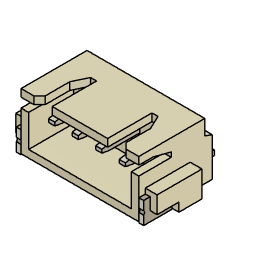
JST-XH SMD Parametric (Autodesk Fusion 360 design; units mm, degrees)
Autodesk Fusion 360 part; units mm, degrees
sketch "Top Ref" plane through (0, 0, 0) normal (0, 0, 1) x (1, 0, 0)
  line L0 (6.25, 0) -> (-6.25, 0)
  line L1 (-6.25, 0) -> (-6.25, -7.8)
  line L2 (-6.25, -7.8) -> (6.25, -7.8)
  line L3 (6.25, -7.8) -> (6.25, 0)
  line L4 (6.25, 0) -> (-6.25, -7.8) construction
  line L5 (-6.25, 0) -> (6.25, -7.8) construction
  line L6 (6.25, -2.35) -> (7.5, -2.35)
  line L7 (7.5, -2.35) -> (7.5, -7.11)
  line L8 (7.5, -7.11) -> (6.25, -7.11)
  line L9 (6.25, -7.11) -> (6.25, -2.35)
  line L10 (0, 0) -> (0, -7.8) construction
  line L11 (-4.07, 0) -> (-4.07, 1.65)
  line L12 (-4.07, 1.65) -> (-3.9378, 2.4)
  line L13 (-3.9378, 2.4) -> (-3.5622, 2.4)
  line L14 (-3.5622, 2.4) -> (-3.43, 1.65)
  line L15 (-3.43, 1.65) -> (-3.43, 0)
  line L16 (-3.75, 2.4) -> (-3.75, 0) construction
  line L17 (-4.07, 1.65) -> (-3.43, 1.65) construction
  line L18 (-6.25, -2.35) -> (-7.5, -2.35)
  line L19 (-7.5, -2.35) -> (-7.5, -7.11)
  line L20 (-7.5, -7.11) -> (-6.25, -7.11)
  line L21 (6.75, -7.11) -> (6.75, -7.8)
  line L22 (6.75, -7.8) -> (6.25, -7.8)
  line L23 (-6.75, -7.11) -> (-6.75, -7.8)
  line L24 (-6.75, -7.8) -> (-6.25, -7.8)
  line L25 (-4.89, -7.8) -> (-4.29, -7.2)
  line L26 (-4.29, -7.2) -> (-4.29, -4.6)
  line L27 (-4.29, -4.6) -> (-3.58, -3.1)
  line L28 (-3.58, -3.1) -> (-2.94, -3.1)
  line L29 (-2.94, -3.1) -> (-2.94, -7.8)
  line L30 (4.89, -7.8) -> (4.29, -7.2)
  line L31 (4.29, -7.2) -> (4.29, -4.6)
  line L32 (4.29, -4.6) -> (3.58, -3.1)
  line L33 (3.58, -3.1) -> (2.94, -3.1)
  line L34 (2.94, -3.1) -> (2.94, -7.8)
  point P0 (0, -3.9)
  point P1 (-3.75, 1.65)
  dimension "d5" = 12.5
  dimension "d6" = 7.5
  dimension "d7" = 4.76
  dimension "d8" = 0.69
  dimension "d9" = 7.8
  dimension "d10" = 0.64
  dimension "d11" = 2.4
  dimension "d12" = 3.75
  dimension "d13" = 80
  dimension "d14" = 0.75
  dimension "d16" = 0.5
  dimension "d17" = 1.35
  dimension "d18" = 4.7
  dimension "d19" = 0.64
  dimension "d20" = 1.5
  dimension "d21" = 45
  dimension "d22" = 1.96
  dimension "d23" = 0.6
  constraint horizontal L0
  constraint perpendicular L0 L1
  constraint parallel L0 L2
  constraint parallel L1 L3
  constraint coincident L4 P0
  constraint coincident L5 P0
  constraint midpoint L10.start L0
  constraint horizontal L6
  constraint vertical L7
  constraint horizontal L8
  constraint vertical L9
  constraint coincident L3 L6.start
  constraint coincident L10.start origin
  constraint midpoint L2 L10.end
  constraint coincident L0 L11.start
  constraint perpendicular L0 L11
  constraint parallel L0 L13
  constraint coincident L0 L15.end
  constraint perpendicular L0 L15
  constraint midpoint L13 L16.start
  constraint coincident L0 L16.end
  constraint perpendicular L0 L16
  constraint horizontal L11.end L14.end
  constraint perpendicular L15 L17
  constraint coincident L16 P1
  constraint midpoint L17 P1
  constraint coincident L1 L18.start
  constraint perpendicular L1 L18
  constraint perpendicular L18 L19
  constraint coincident L1 L20.end
  constraint perpendicular L1 L20
  constraint equal L6 L18
  constraint equal L7 L19
  constraint horizontal L8.end L20.end
  constraint coincident L8 L21.start
  constraint perpendicular L8 L21
  constraint perpendicular L21 L22
  constraint coincident L20 L23.start
  constraint perpendicular L20 L23
  constraint perpendicular L23 L24
  constraint equal L22 L24
  constraint coincident L2 L25.start
  constraint perpendicular L2 L26
  constraint perpendicular L26 L28
  constraint coincident L2 L29.end
  constraint perpendicular L2 L29
  constraint symmetric L10 L25.start L30.start
  constraint symmetric L10 L25.end L30.end
  constraint symmetric L10 L26.end L31.end
  constraint symmetric L10 L27.end L32.end
  constraint symmetric L10 L28.end L33.end
  constraint symmetric L10 L29.end L34.end
  constraint coincident L2.end L3.start
  constraint coincident L1.end L2.start
  measures "d5" distance of L1.end L2.end
  measures "d6" distance of L10.start L7
  measures "d7" distance of L6.end L7.end
  measures "d8" distance of L2.end L8
  measures "d9" distance of L0.end L1.end
  measures "d10" distance of L11.end L14.end
  measures "d11" distance of L16.start L16.end
  measures "d12" distance of L10.start L16.end
  measures "d13" angle of L14 L17
  measures "d14" distance of L13 L14.end
  measures "d16" distance of L21.end L2.end
  measures "d17" distance of L26 L29
  measures "d18" distance of L2 L28
  measures "d19" distance of L27.end L28.end
  measures "d20" distance of L26.end L28
  measures "d21" angle of L2 L25
  measures "d22" distance of L1 L26
  measures "d23" distance of L2 L25.end
sketch "Side Ref" plane through (0, 0, 0) normal (1, 0, 0) x (0, 1, 0)
  line L0 (0, 0) -> (0, 6)
  line L1 (0, 6) -> (-7.8, 6)
  line L2 (-7.8, 6) -> (-7.8, 0)
  line L3 (-7.8, 0) -> (0, 0)
  line L4 (0, 4.1) -> (-0.8, 4.395)
  line L5 (-0.8, 4.395) -> (-0.8, 6)
  line L6 (-0.8, 5.47) -> (-1.33, 5.47)
  line L7 (-1.33, 5.47) -> (-1.33, 4.395)
  line L8 (-1.33, 4.395) -> (-0.9, 4.395)
  line L9 (-0.9, 4.395) -> (-0.9, 3.145)
  line L10 (-0.9, 3.145) -> (-1.5, 3.145)
  line L11 (-1.5, 3.145) -> (-1.5, 1.12)
  line L12 (-1.5, 1.12) -> (0, 1.12)
  line L13 (-7.8, 5.2) -> (-3.03, 5.2)
  line L14 (-6.3, 5.2) -> (-4.35, 4.7)
  line L15 (-4.35, 4.7) -> (-4.35, 4.2)
  line L16 (-4.35, 4.2) -> (-7.8, 4.2)
  line L17 (-3.03, 5.2) -> (-3.03, 0.8)
  line L18 (-3.03, 0.8) -> (-7.8, 0.8)
  line L19 (-4.35, 4.7) -> (-4.35, 5.2) construction
  line L20 (-3.03, 4.09) -> (-6.25, 4.09)
  line L21 (-6.25, 4.09) -> (-7.05, 3.9489)
  line L22 (-7.05, 3.9489) -> (-7.05, 3.5911)
  line L23 (-7.05, 3.5911) -> (-6.25, 3.45)
  line L24 (-6.25, 3.45) -> (-3.03, 3.45)
  line L25 (-7.05, 3.77) -> (-3.03, 3.77) construction
  point P0 (-1.065, 5.47)
  point P1 (-0.9, 3.77)
  dimension "d24" = 6
  dimension "d25" = 7.8
  dimension "d26" = 7
  dimension "d27" = 1.9
  dimension "d29" = 1.12
  dimension "d30" = 1.5
  dimension "d31" = 0.53
  dimension "d32" = 0.53
  dimension "d34" = 1.25
  dimension "d36" = 0.1
  dimension "d60" = 0.8
  dimension "d61" = 0.8
  dimension "d62" = 4.77
  dimension "d63" = 3.45
  dimension "d64" = 1.5
  dimension "d65" = 1
  dimension "d66" = 0.8
  dimension "d67" = 10
  dimension "d68" = 0.64
  dimension "d69" = 0.75
  dimension "d70" = 2.55
  constraint coincident L0.start L3.end
  constraint vertical L0
  constraint perpendicular L0 L1
  constraint perpendicular L1 L2
  constraint horizontal L3
  constraint coincident L0 L4.start
  constraint coincident L1 L5.end
  constraint perpendicular L1 L5
  constraint coincident L5 L6.start
  constraint perpendicular L5 L6
  constraint perpendicular L6 L7
  constraint perpendicular L7 L8
  constraint perpendicular L8 L9
  constraint perpendicular L7 L10
  constraint perpendicular L3 L11
  constraint coincident L0 L12.end
  constraint perpendicular L0 L12
  constraint midpoint L6 P0
  constraint horizontal L4.end L8.end
  constraint coincident L2 L13.start
  constraint perpendicular L2 L13
  constraint perpendicular L13 L15
  constraint coincident L2 L16.end
  constraint perpendicular L2 L16
  constraint perpendicular L13 L17
  constraint coincident L2 L18.end
  constraint perpendicular L2 L18
  constraint coincident L14.start L13
  constraint coincident L13 L19.end
  constraint perpendicular L13 L19
  constraint equal L15 L19
  constraint coincident L17 L20.start
  constraint perpendicular L17 L20
  constraint perpendicular L20 L22
  constraint coincident L17 L24.end
  constraint perpendicular L17 L24
  constraint midpoint L22 L25.start
  constraint coincident L17 L25.end
  constraint perpendicular L17 L25
  constraint vertical L20.end L23.end
  constraint equal L21 L23
  constraint midpoint L9 P1
  constraint horizontal L25.end P1
  measures "d24" distance of L0.start L0.end
  measures "d25" distance of L0.end L1.end
  measures "d26" distance of L1.end L5.end
  measures "d27" distance of L0.end L4.start
  measures "d29" distance of L12 L0.start
  measures "d30" distance of L11.end L12.end
  measures "d31" distance of L1 L6
  measures "d32" distance of L6.start L6.end
  measures "d34" distance of L8.end L9.end
  measures "d36" distance of L4.end L8.end
  measures "d60" distance of L1 L13
  measures "d61" distance of L3 L18
  measures "d62" distance of L13.start L13.end
  measures "d63" distance of L15.end L16.end
  measures "d64" distance of L13.start L14.start
  measures "d65" distance of L13 L16
  measures "d66" horizontal distance of L20.end L21.end
  measures "d67" angle of L20 L21
  measures "d68" distance of L20 L24
  measures "d69" distance of L2 L25.start
  measures "d70" distance of L1 L23.end
extrude "Extrude1" add sketch "Side Ref" along normal mid plane 12.5 contours L0 L1 L2 L3 L5 L6 L7 L8 L9 L10 L11 L12 L13 L17 L18 | L2 L13 L14 L15 L16 L17 L18 L20 L21 L22 L23 L24 | L2 L13 L14 L15 L16 | L17 L20 L21 L22 L23 L24 makes body 1
ref_plane "WorkPlane1" through (-3.75, 1.2, 0) normal (-1, 0, 0) x (0, -1, 0)
extrude "Extrude2" add sketch "Side Ref" against normal blind 0.82 from surface at 6.25 contours L0 L1 L2 L3 L5 L6 L7 L8 L9 L10 L11 L12 L13 L17 L18 | L0 L4 L5 L6 L7 L8 L9 L10 L11 L12 | L2 L13 L14 L15 L16 L17 L18 L20 L21 L22 L23 L24 | L2 L13 L14 L15 L16 | L17 L20 L21 L22 L23 L24 bodies 1
extrude "Extrude3" add sketch "Side Ref" along normal blind 0.82 from surface at -6.25 contours L0 L1 L2 L3 L5 L6 L7 L8 L9 L10 L11 L12 L13 L17 L18 | L0 L4 L5 L6 L7 L8 L9 L10 L11 L12 | L2 L13 L14 L15 L16 L17 L18 L20 L21 L22 L23 L24 | L2 L13 L14 L15 L16 | L17 L20 L21 L22 L23 L24 bodies 1
extrude "Extrude6" cut sketch "Side Ref" along normal mid plane 10.9 contours L2 L13 L14 L15 L16 L17 L18 L20 L21 L22 L23 L24 | L2 L13 L14 L15 L16 | L17 L20 L21 L22 L23 L24 bodies 1
extrude "Extrude7" cut sketch "Side Ref" along normal mid plane 12.5 contours L2 L13 L14 L15 L16 bodies 1
extrude "Extrude8" cut sketch "Top Ref" along normal blind 6 from surface at 1 contours L2 L30 L31 L32 L33 L34 | L2 L25 L26 L27 L28 L29 bodies 1
sketch "Pin Side" plane through (-3.75, 0, 0) normal (-1, 0, 0) x (0, -1, 0)
  line L0 (-2.4, 0) -> (0, 0) construction
  line L1 (-2.4, -0.1) -> (0.64, -0.1)
  line L2 (-2.4, -0.1) -> (-2.4, 0.54)
  line L3 (-2.4, 0.54) -> (0, 0.54)
  line L4 (0.64, -0.1) -> (0.64, 3.45)
  line L5 (0, 0.54) -> (0, 4.09)
  line L6 (0.9, 4.395) -> (0.9, 3.145) construction
  line L7 (0.9, 4.09) -> (0.9, 3.45)
  line L8 (0.9, 4.09) -> (0, 4.09)
  line L9 (0.9, 3.45) -> (0.64, 3.45)
  line L10 (0.64, 3.45) -> (0, 3.45) construction
  line L11 (-2.4, 0.4078) -> (-1.65, 0.54)
  arc A0 (0.2, 4.09) -> (0, 3.89) centre (0.2, 3.89) ccw
  arc A1 (-0.1, 0.54) -> (0, 0.64) centre (-0.1, 0.64) ccw
  line L12 (6.25, 4.09) -> (7.05, 3.9489)
  line L13 (7.05, 3.9489) -> (7.05, 3.5911)
  line L14 (7.05, 3.5911) -> (6.25, 3.45)
  line L15 (6.25, 3.45) -> (3.03, 3.45)
  line L16 (3.03, 4.09) -> (6.25, 4.09)
  line L17 (3.03, 4.09) -> (3.03, 3.45)
  line L18 (3.03, 4.09) -> (0.9, 4.09)
  line L19 (3.03, 3.45) -> (0.9, 3.45)
  point P0 (0.9, 3.77)
  point P1 (-1.65, 0)
  dimension "d46" = 0.1
  dimension "d47" = 0.64
  dimension "d48" = 10
  dimension "d49" = 0.2
  dimension "d50" = 0.1
  constraint horizontal L1
  constraint vertical L0.start L1.start
  constraint perpendicular L0 L2
  constraint perpendicular L2 L3
  constraint perpendicular L1 L4
  constraint perpendicular L3 L5
  constraint midpoint L6 P0
  constraint coincident L6 L7.start
  constraint coincident L6 L7.end
  constraint parallel L6 L7
  constraint midpoint P0 L7
  constraint horizontal L8
  constraint horizontal L9
  constraint equal L2 L7
  constraint coincident L5 L10.end
  constraint perpendicular L5 L10
  constraint equal L2 L10
  constraint vertical L3.end L0.end
  constraint coincident L2 L11.start
  constraint coincident L3 L11.end
  constraint vertical P1 L11.end
  constraint tangent L8 A0
  constraint coincident L5 A0.end
  constraint coincident L8 A0.start
  constraint tangent L5 A0
  constraint coincident L3 A1.start
  constraint coincident L5 A1.end
  constraint tangent L5 A1
  constraint tangent L3 A1
  constraint coincident L16.start L17.start
  constraint coincident L15.end L17.end
  constraint coincident L7.start L8.start
  constraint coincident L7.end L9.start
  measures "d46" distance of L0.start L1.start
  measures "d47" distance of L1.start L2.end
  measures "d48" angle of L3 L11
  measures "d49" radius of A0
  measures "d50" radius of A1
extrude "Extrude4" cut sketch "Pin Side" along normal mid plane 0.66 contours L1 L2 L3 L4 L5 L7 L8 L9 L11 A0 | L7 L17 L18 L19 | L3 L5 A1 | L12 L13 L14 L15 L16 L17 | L5 L8 A0 bodies 1
extrude "Extrude5" add sketch "Pin Side" along normal mid plane 0.65 separate body contours L1 L2 L3 L4 L5 L7 L8 L9 L11 A0 | L7 L17 L18 L19 | L3 L5 A1 | L12 L13 L14 L15 L16 L17 makes body 2
pattern_linear "R-Pattern1" count 4 spacing 2.5 along (1, 0, 0) of "Extrude4"
pattern_linear "R-Pattern3" count 4 spacing 2.5 along (1, 0, 0) of bodies 2 makes body 3 at (-1.575, -2.3633, 3.8767) makes body 4 at (0.925, -2.3633, 3.8767) makes body 5 at (3.425, -2.3633, 3.8767)
sketch "Side Anchors" plane through (0, 0, 0) normal (1, 0, 0) x (0, 1, 0)
  line L0 (-7.8, 6) -> (-7.8, 0) construction
  line L1 (-7.8, 0) -> (0, 0) construction
  line L2 (-2.35, 0) -> (-2.35, 2.75)
  line L3 (-2.35, 2.75) -> (-7.11, 2.75)
  line L4 (-7.11, 2.75) -> (-7.11, 0.93)
  line L5 (-7.11, 0.93) -> (-4.8, 0.93)
  line L6 (-7.8, -0.1) -> (-7.8, 2.21)
  line L7 (-7.8, 2.21) -> (-4.8, 2.21)
  line L8 (-4.8, 2.21) -> (-4.8, -0.1)
  line L9 (-4.8, -0.1) -> (-7.8, -0.1)
  line L10 (-2.35, 0) -> (-4.8, 0)
  arc A0 (-7.8, 0.855) -> (-7.8, 1.255) centre (-7.95, 1.055) ccw
  point P0 (-7.8, 0)
  point P1 (-7.11, 0)
  point P2 (-2.35, 0)
  point P3 (-7.8, 1.055)
  dimension "d79" = 2.75
  dimension "d80" = 1.82
  dimension "d81" = 2.31
  dimension "d82" = 0.1
  dimension "d83" = 3
  dimension "d95" = 0.25
  dimension "d96" = 0.15
  constraint coincident P2 L2.start
  constraint perpendicular L1 L2
  constraint perpendicular L0 L3
  constraint perpendicular L3 L4
  constraint perpendicular L0 L5
  constraint vertical P1 L4.end
  constraint vertical L6
  constraint perpendicular L0 L7
  constraint perpendicular L7 L8
  constraint perpendicular L8 L9
  constraint coincident L6.start L9.end
  constraint coincident L5.end L8
  constraint coincident L8 L10.end
  constraint coincident L1 L10.end
  constraint coincident P0 L6
  constraint coincident L0 A0.start
  constraint coincident L6 P3
  constraint midpoint L6 P3
  constraint horizontal A0.centre P3
  constraint coincident L6 A0.end
  measures "d79" distance of P2 L2.end
  measures "d80" distance of L3.end L4.end
  measures "d81" distance of L6.start L6.end
  measures "d82" vertical distance of P0 L6.start
  measures "d83" distance of L8.end L6.start
  measures "d95" radius of A0
  measures "d96" distance of A0.centre P3
extrude "Extrude9" add sketch "Side Anchors" along normal blind 1.25 from surface at 6.25 contours L2 L3 L4 L7 L8 L10 | L4 L5 L7 L8 bodies 1 2
extrude "Extrude10" cut sketch "Side Anchors" along normal blind 0.52 from surface at 6.25 contours L4 L5 L6 L7 L8 L9 A0 | L4 L5 L7 L8 | L6 A0 bodies 2 1
extrude "Extrude11" add sketch "Side Anchors" along normal blind 0.5 from surface at 6.26 separate body contours L4 L5 L6 L7 L8 L9 A0 | L4 L5 L7 L8 makes body 6
mirror "Mirror1" about plane through (0, 0, 0) normal (1, 0, 0) of "Extrude9", "Extrude10"
mirror "Mirror3" about plane through (0, 0, 0) normal (1, 0, 0) of bodies 6 makes body 7
ref_plane "WorkPlane2" through (-3.75, 0.88, -0.1) normal (0, 0, 1) x (0, -1, 0)
sketch "Footprint Reference" plane through (0, 0, -0.1) normal (0, 0, 1) x (1, 0, 0)
  line L0 (6.25, -7.8) -> (6.25, 0) construction
  line L1 (6.25, 0) -> (-6.25, 0) construction
  line L2 (-6.25, -7.8) -> (6.25, -7.8) construction
  line L3 (-6.25, 0) -> (-6.25, -7.8) construction
  line L4 (6.26, -7.8) -> (6.26, -4.8) construction
  line L5 (6.26, -4.8) -> (6.76, -4.8) construction
  line L6 (6.76, -4.8) -> (6.76, -7.8) construction
  line L7 (6.76, -7.8) -> (6.26, -7.8) construction
  line L8 (-6.26, -4.8) -> (-6.26, -7.8) construction
  line L9 (-6.26, -7.8) -> (-6.76, -7.8) construction
  line L10 (-6.76, -7.8) -> (-6.76, -4.8) construction
  line L11 (-6.76, -4.8) -> (-6.26, -4.8) construction
  line L12 (-3.425, -0.64) -> (-4.075, -0.64) construction
  line L13 (-4.075, -0.64) -> (-4.075, 2.4) construction
  line L14 (-4.075, 2.4) -> (-3.425, 2.4) construction
  line L15 (-3.425, 2.4) -> (-3.425, -0.64) construction
  line L16 (-3.225, -0.84) -> (-4.275, -0.84)
  line L17 (-4.275, -0.84) -> (-4.275, 2.6)
  line L18 (-4.275, 2.6) -> (-3.225, 2.6)
  line L19 (-3.225, 2.6) -> (-3.225, -0.84)
  line L20 (-6.06, -8) -> (-6.96, -8)
  line L21 (-6.96, -8) -> (-6.96, -4.6)
  line L22 (-6.96, -4.6) -> (-6.06, -4.6)
  line L23 (-6.06, -4.6) -> (-6.06, -8)
  line L24 (6.96, -8) -> (6.06, -8)
  line L25 (6.06, -8) -> (6.06, -4.6)
  line L26 (6.06, -4.6) -> (6.96, -4.6)
  line L27 (6.96, -4.6) -> (6.96, -8)
  line L28 (-4.275, 2.6) -> (-3.225, -0.84) construction
  line L29 (-3.225, 2.6) -> (-4.275, -0.84) construction
  line L30 (-6.96, -4.6) -> (-6.06, -8) construction
  line L31 (-6.96, -8) -> (-6.06, -4.6) construction
  line L32 (6.96, -4.6) -> (6.06, -8) construction
  line L33 (6.96, -8) -> (6.06, -4.6) construction
  line L34 (-0.725, -0.84) -> (-1.775, -0.84)
  line L35 (-1.775, -0.84) -> (-1.775, 2.6)
  line L36 (-0.725, 2.6) -> (-0.725, -0.84)
  line L37 (-1.775, 2.6) -> (-0.725, 2.6)
  line L38 (-0.725, 2.6) -> (-1.775, -0.84) construction
  line L39 (-1.775, 2.6) -> (-0.725, -0.84) construction
  line L40 (1.775, -0.84) -> (0.725, -0.84)
  line L41 (0.725, -0.84) -> (0.725, 2.6)
  line L42 (1.775, 2.6) -> (1.775, -0.84)
  line L43 (0.725, 2.6) -> (1.775, 2.6)
  line L44 (1.775, 2.6) -> (0.725, -0.84) construction
  line L45 (0.725, 2.6) -> (1.775, -0.84) construction
  line L46 (4.275, -0.84) -> (3.225, -0.84)
  line L47 (3.225, -0.84) -> (3.225, 2.6)
  line L48 (4.275, 2.6) -> (4.275, -0.84)
  line L49 (3.225, 2.6) -> (4.275, 2.6)
  line L50 (4.275, 2.6) -> (3.225, -0.84) construction
  line L51 (3.225, 2.6) -> (4.275, -0.84) construction
  point P0 (-3.75, 0.88)
  point P1 (-6.51, -6.3)
  point P2 (6.51, -6.3)
  point P3 (-1.25, 0.88)
  point P4 (1.25, 0.88)
  point P5 (3.75, 0.88)
  point P6 (0, -3.9)
  dimension "d118" = 2.5
  dimension "d119" = 0
  dimension "d133" = 0.9
  dimension "d134" = 3.4
  dimension "d135" = 7.8
  dimension "d136" = 12.5
  dimension "d137" = 3.75
  dimension "d138" = 4.78
  dimension "d139" = 1.25
  dimension "d140" = 1.25
  dimension "d141" = 3.75
  dimension "d144" = 6.51
  dimension "d145" = 2.4
  dimension "d147" = 1.05
  dimension "d148" = 3.44
  constraint coincident L28 P0
  constraint coincident L29 P0
  constraint coincident L31 P1
  constraint coincident L30 P1
  constraint coincident L33 P2
  constraint coincident L32 P2
  measures "d133" distance of L25.end L26.end
  measures "d134" distance of L24.start L26.end
  measures "d135" distance of L1.end L2.start
  measures "d136" distance of L0.start L2.start
  measures "d137" horizontal distance of P0 P6
  measures "d138" vertical distance of P0 P6
  measures "d139" horizontal distance of P3 P6
  measures "d140" horizontal distance of P4 P6
  measures "d141" horizontal distance of P5 P6
  measures "d144" horizontal distance of P1 P6
  measures "d145" vertical distance of P1 P6
  measures "d147" distance of L17.end L18.end
  measures "d148" distance of L16.end L17.end
equation "Pin_Qty = 4" comment "Yes Touchy"
equation "Pin_Extent_A = Pin_Spacing * ( Pin_Qty - 1 )" comment "No Touchy"
equation "Width_B = ( Pin_Spacing * Pin_Qty ) + Pin_Spacing" comment "No Touchy"
equation "Width_C = ( Pin_Spacing * Pin_Qty ) + 2 * Pin_Spacing" comment "No Touchy"
equation "d5 = Width_B"
equation "d6 = Width_C / 2"
equation "d12 = Pin_Extent_A / 2"
equation "d37 = Width_B"
equation "d40 = Width_B / 2"
equation "d43 = -Width_B / 2"
equation "d48 = 90 deg - 80 deg"
equation "d56 = Pin_Qty"
equation "d58 = -Pin_Spacing"
equation "d71 = Width_B / 2 - 0.8 mm"
equation "d73 = Width_B"
equation "d84 = Width_B / 2"
equation "d85 = ( Width_C - Width_B ) / 2"
equation "d89 = Width_B / 2"
equation "d92 = Width_B / 2 + 0.01 mm"
equation "Pin_Spacing = 2.5 mm" comment "No Touchy"
equation "d104 = Pin_Qty"
equation "d106 = Pin_Spacing"
equation "SMD_Pad_Expansion = 0.2 mm" comment "No Touchy"
equation "d113 = -SMD_Pad_Expansion"
equation "d114 = -SMD_Pad_Expansion"
equation "d115 = -SMD_Pad_Expansion"
equation "d116 = Pin_Qty"
equation "d118 = Pin_Spacing"
named bodies: "Connector body", "Anchor Plate", "Pin", "Pin (1)", "Anchor Plate (1)", "Pin (2)", "Pin (3)"
